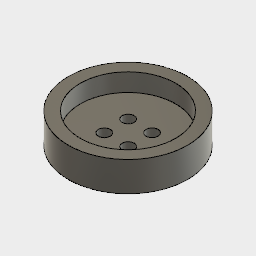
kouzi v1 (Autodesk Fusion 360 design; units mm, degrees)
Autodesk Fusion 360 part; units mm, degrees
sketch "草图1" plane through (0, 0, 0) normal (0, 1, 0) x (1, 0, 0)
  circle A0 centre (0, 0) radius 10
  circle A1 centre (0, 0) radius 8
  dimension "d2" = 2
surface "拉伸1" add extruded along (0, 1, 0) between 0 and 2 profiles "草图1" section 1 contours A1 makes body 1
extrude "拉伸2" add sketch "草图1" along normal blind 2 separate body contours A1 makes body 2
extrude "拉伸3" add sketch "草图1" along normal blind 5 bodies 2
cylinder "圆柱体基本要素1" add diameter 2 height 20 placed x (1, 0, 0) y (0, 0, -1) z (0, 1, 0) at (15, 0, -5) separate body makes body 3
move_face "MoveFace1" to x (1, 0, 0) y (0, 1, 0) z (0, 0, 1) at (-12.7881, 0, 7.1797) 1 faces at (15.995, 13.3333, -4.9004) on bodies 3
pattern_linear "R-阵列1" count 1 spacing 0 along (0, 0, 1) count 2 spacing 4 along (-1, 0, 0) of bodies 3 makes body 4
pattern_linear "R-阵列2" count 1 spacing 0 along (1, 0, 0) count 2 spacing 4 along (0, 0, -1) of bodies 4 3 makes body 5 at (-0.7931, 13.3333, -1.7207) makes body 6 at (3.2069, 13.3333, -1.7207)
combine "合并1" operation cut target body 2 tool bodies 6 5 4 3
hidden bodies 1
